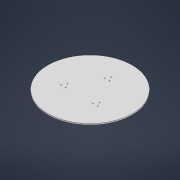
# Autodesk Inventor part: Table
Saved by Autodesk Inventor 2023 (Build 270158000, 158)
## iProperties
Created: 2022-05-02
Part Number: Table
Material: Generic
Document SubType Name: Modeling
Designer: FizzyApple12
Density: 1 g/cm^3
Appearance: Default
Author: FizzyApple12
Autodesk Inventor part; units mm, degrees
ref_plane "YZ Plane" through (0, 0, 0) normal (1, 0, 0) x (0, 1, 0)
ref_plane "XZ Plane" through (0, 0, 0) normal (0, 1, 0) x (-1, 0, 0)
ref_plane "XY Plane" through (0, 0, 0) normal (0, 0, 1) x (1, 0, 0)
sketch "Sketch1" plane through (0, 0, 0) normal (0, 1, 0) x (-1, 0, 0)
  circle A0 centre (0, 0) radius 228.6
  line L0 (228.6, 0) -> (-228.6, 0) construction
  line L1 (0, -115.0592) -> (-99.6442, 57.5296) construction
  line L2 (-99.6442, 57.5296) -> (99.6442, 57.5296) construction
  line L3 (99.6442, 57.5296) -> (0, -115.0592) construction
  line L4 (99.6442, 57.5296) -> (74.2442, 57.5296) construction
  line L5 (99.6442, 57.5296) -> (86.9442, 35.5326) construction
  line L6 (-99.6442, 57.5296) -> (-74.2442, 57.5296) construction
  line L7 (-99.6442, 57.5296) -> (-86.9442, 35.5326) construction
  line L8 (0, -115.0592) -> (12.7, -93.0622) construction
  line L9 (0, -115.0592) -> (-12.7, -93.0622) construction
  dimension "d26" = 457.2
  dimension "d27" = 199.2884
  dimension "d28" = 25.4
  dimension "d29" = 25.4
  dimension "d30" = 25.4
  dimension "d31" = 25.4
  dimension "d32" = 25.4
  dimension "d33" = 25.4
  constraints: 20 end point, 11 coincident, 6 point on line, 2 point on circle, 1 centre point, 1 horizontal, 1 midpoint, 1 parallel, 7 other
  measures "d26" diameter of A0
  measures "d27" distance of L1.end L2.end
  measures "d28" distance of L4.start L4.end
  measures "d29" distance of L4.start L5.end
  measures "d30" distance of L6.start L6.end
  measures "d31" distance of L6.start L7.end
  measures "d32" distance of L8.start L8.end
  measures "d33" distance of L8.start L9.end
extrude "Extrusion1" add sketch "Sketch1" along normal blind 6.35
hole "Hole1" at (-99.6442, 0, 57.5296) at (-74.2442, 0, 57.5296) at (-86.9442, 0, 35.5326) at (-12.7, 0, -93.0622) at (0, 0, -115.0592) at (12.7, 0, -93.0622) at (99.6442, 0, 57.5296) at (74.2442, 0, 57.5296) at (86.9442, 0, 35.5326) direction (0, 1, 0) diameter 3.9624 end through all thread size "10-32 UNF" class "2B" standard "ANSI Unified Screw Threads"
body "Solid1"
